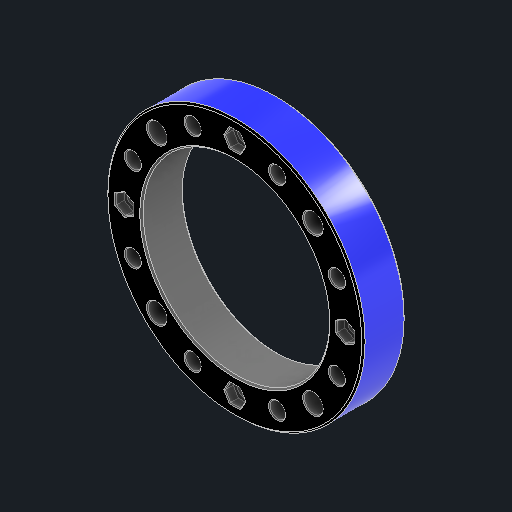
# Autodesk Inventor part: CF150-spacer
Saved by Autodesk Inventor 2025 (Build 290162000, 162)
## iProperties
Created: 2024-05-24
Part Number: CF150-spacer
Material: PET Plastic
Document SubType Name: Modeling
Designer: kuzmin
Density: 1.541 g/cm^3
Appearance: Gray
Author: kuzmin
Autodesk Inventor part; units mm, degrees
ref_plane "YZ Plane" through (0, 0, 0) normal (1, 0, 0) x (0, 1, 0)
ref_plane "XZ Plane" through (0, 0, 0) normal (0, 1, 0) x (-1, 0, 0)
ref_plane "XY Plane" through (0, 0, 0) normal (0, 0, 1) x (1, 0, 0)
sketch "Sketch1" plane through (0, 0, 0) normal (0, 0, 1) x (1, 0, 0)
  circle A0 centre (0, 0) radius 75.8
  dimension "d0" = 151.6
  constraints: 1 centre point, 1 coincident
  measures "d0" diameter of A0
extrude "Extrusion1" add sketch "Sketch1" along normal blind 25
sketch "Sketch2" plane through (0, 0, 25) normal (0, 0, 1) x (1, 0, 0)
  circle A0 centre (0, 0) radius 55
  dimension "d3" = 110
  constraints: 1 centre point, 1 coincident
  measures "d3" diameter of A0
extrude "Extrusion2" cut sketch "Sketch2" against normal through all
sketch "Sketch3" plane through (0, 0, 25) normal (0, 0, 1) x (1, 0, 0)
  circle A0 centre (0, 0) radius 65.125 construction
  point P0 (65.125, 0)
  dimension "d6" = 130.25
  constraints: 2 horizontal alignment, 1 coincident, 2 other
hole "Hole1" at (65.125, 0, 25) direction (0, 0, -1) diameter 9 end through all
chamfer "Chamfer2" distance 0.5 angle 45 2 edges at (65.125, 4.5, 25) (65.125, 4.5, 0)
pattern_circular "Circular Pattern1" count 16 over 360 about axis through (0, 0, 0) along (0, 0, 1) of "Hole1", "Chamfer2"
chamfer "Chamfer1" distance 1 angle 45 4 edges at (-75.8, 0, 25) (-75.8, 0, 0) (-55, 0, 25) (-55, 0, 0)
sketch "Sketch4" plane through (0, 0, 25) normal (0, 0, 1) x (1, 0, 0)
  circle A0 centre (0, 65.125) radius 4.5 projected
  line L0 (-2.9734, 59.975) -> (-5.9467, 65.125)
  line L1 (-5.9467, 65.125) -> (-2.9734, 70.275)
  line L2 (-2.9734, 70.275) -> (2.9734, 70.275)
  line L3 (2.9734, 70.275) -> (5.9467, 65.125)
  line L4 (5.9467, 65.125) -> (2.9734, 59.975)
  line L5 (2.9734, 59.975) -> (-2.9734, 59.975)
  point P0 (0, 0)
  dimension "d23" = 10.3
  constraints: 12 end point, 1 coincident, 1 horizontal, 13 other
  measures "d23" distance between parallel lines of L5 L2
extrude "Extrusion3" cut sketch "Sketch4" against normal blind 5
sketch "Sketch5" plane through (0, 0, 20) normal (0, 0, 1) x (1, 0, 0)
  circle A0 centre (0, 65.125) radius 4.5 projected
  circle A1 centre (0, 65.125) radius 3.25
  point P0 (0, 0)
  dimension "d26" = 6.5
  constraints: 1 centre point, 1 coincident
  measures "d26" diameter of A1
extrude "Extrusion4" add sketch "Sketch5" against normal blind 19.5
sketch "Sketch6" plane through (0, 0, 0) normal (0, 0, -1) x (-1, 0, 0)
  circle A0 centre (0, 65.125) radius 5 projected
  circle A1 centre (0, 65.125) radius 3.25 projected
  point P0 (0, 0)
extrude "Extrusion5" add sketch "Sketch6" against normal up to surface (0.5 mm away)
chamfer "Chamfer4" distance 0.5 angle 45 6 edges at (0, 59.975, 25) (-4.46, 62.55, 25) (-4.46, 67.7, 25) (0, 70.275, 25) (4.46, 67.7, 25) (4.46, 62.55, 25)
pattern_circular "Circular Pattern2" count 4 over 360 about axis through (0, 0, 0) along (0, 0, 1) of "Extrusion5", "Extrusion4", "Extrusion3", "Chamfer4"
sketch "Sketch7" plane through (0, 0, 25) normal (0, 0, 1) x (1, 0, 0)
  circle A0 centre (46.0503, 46.0503) radius 5 projected
  circle A1 centre (46.0503, 46.0503) radius 3.25
  point P0 (0, 0)
  dimension "d37" = 6.5
  constraints: 1 centre point, 1 coincident
  measures "d37" diameter of A1
extrude "Extrusion6" add sketch "Sketch7" against normal up to surface (25 mm away)
sketch "Sketch8" plane through (0, 0, 25) normal (0, 0, 1) x (1, 0, 0)
  circle A0 centre (46.0503, 46.0503) radius 3.25 projected
  circle A1 centre (46.0503, 46.0503) radius 5.5
  point P0 (0, 0)
  dimension "d40" = 11
  constraints: 1 centre point, 1 coincident
  measures "d40" diameter of A1
extrude "Extrusion7" cut sketch "Sketch8" against normal blind 8
chamfer "Chamfer5" distance 0.5 angle 45 1 edges at (40.5503, 46.0503, 25)
pattern_circular "Circular Pattern3" count 4 over 360 about axis through (0, 0, 0) along (0, 0, 1) of "Extrusion6", "Extrusion7", "Chamfer5"
sketch "Sketch9" plane through (0, 0, 0) normal (0, 0, -1) x (-1, 0, 0)
  circle A0 centre (-65.125, 0) radius 3.25 projected
  circle A1 centre (-65.125, 0) radius 6.1
  point P0 (0, 0)
  dimension "d46" = 12.2
  constraints: 1 centre point, 1 coincident
  measures "d46" diameter of A1
extrude "Extrusion8" cut sketch "Sketch9" against normal blind 10
sketch "Sketch10" plane through (65.125, 0, 10) normal (0, 0, -1) x (-1, 0, 0)
  circle A0 centre (0, 0) radius 6.1 projected
  line L0 (3.25, 5.1621) -> (-3.25, 5.1621)
  line L1 (-3.25, 5.1621) -> (-3.25, -5.1621)
  line L2 (-3.25, -5.1621) -> (3.25, -5.1621)
  line L3 (3.25, -5.1621) -> (3.25, 5.1621)
  circle A1 centre (0, 0) radius 3.25 projected
  point P0 (65.125, 0)
  point P1 (3.25, -5.1621)
  constraints: 8 end point, 2 parallel, 2 point on circle, 2 tangent, 1 horizontal, 1 perpendicular
extrude "Extrusion9" add sketch "Sketch10" along normal blind 0.6 contours A0 L3 | L1 A0
sketch "Sketch11" plane through (0, 0, 10) normal (0, 0, -1) x (-1, 0, 0)
  circle A0 centre (-65.125, 0) radius 6.1 projected
  arc A1 (-68.375, 0) -> (-61.875, 0) centre (-65.125, 0) ccw projected
  arc A2 (-61.875, 0) -> (-68.375, 0) centre (-65.125, 0) ccw projected
  line L0 (-59.9629, 3.25) -> (-70.2871, 3.25)
  line L1 (-70.2871, 3.25) -> (-70.2871, -3.25)
  line L2 (-70.2871, -3.25) -> (-59.9629, -3.25)
  line L3 (-59.9629, -3.25) -> (-59.9629, 3.25)
  point P0 (0, 0)
  constraints: 8 end point, 2 parallel, 2 point on circle, 2 tangent, 1 horizontal, 1 perpendicular
extrude "Extrusion10" add sketch "Sketch11" along normal blind 0.3 contours L0 A0 | A0 L2
chamfer "Chamfer6" distance 0.5 angle 45 1 edges at (71.225, 0, 0)
pattern_circular "Circular Pattern4" count 8 over 360 about axis through (0, 0, 0) along (0, 0, 1) of "Extrusion8", "Extrusion9", "Extrusion10", "Chamfer6"
body "Solid1"
